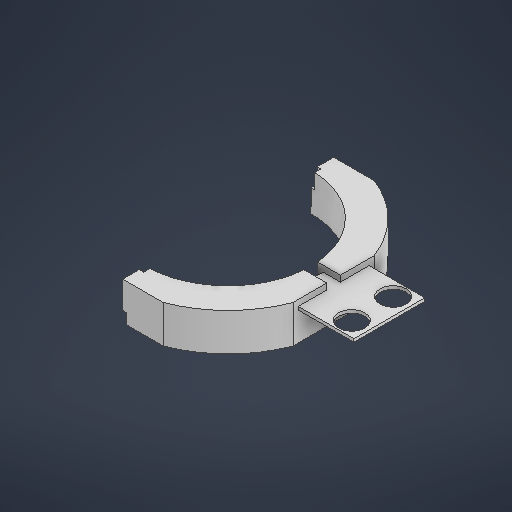
# Autodesk Inventor part: Kruh
Saved by Autodesk Inventor 2026.2 (Build 302298000, 298)
## iProperties
Created: 2026-03-13
Part Number: Kruh
Material: Všeobecné
Document SubType Name: Modeling
Designer: cerna
Density: 1 g/cm^3
Appearance: Výchozí
Author: cerna
Autodesk Inventor part; units mm, degrees
sketch "Náčrt1" plane through (0, 0, 0) normal (0, 1, 0) x (-1, 0, 0)
  circle A0 centre (0, 0) radius 55
  line L0 (0, -70) -> (26.9258, -70)
  line L1 (0, -70) -> (-26.9258, -70)
  line L2 (-70, 0) -> (-70, -26.9258)
  line L3 (-70, 0) -> (-70, 26.9258)
  line L4 (70, 0) -> (70, -26.9258)
  line L5 (70, 0) -> (70, 26.9258)
  line L6 (0, 70) -> (26.9258, 70)
  line L7 (0, 70) -> (-26.9258, 70)
  line L8 (-104.3981, 0) -> (104.3981, 0) projected
  line L9 (0, -104.3981) -> (0, 104.3981) projected
  arc A1 (26.9258, -70) -> (70, -26.9258) centre (0, 0) ccw
  arc A2 (-70, -26.9258) -> (-26.9258, -70) centre (0, 0) ccw
  arc A3 (70, 26.9258) -> (26.9258, 70) centre (0, 0) ccw
  arc A4 (-26.9258, 70) -> (-70, 26.9258) centre (0, 0) ccw
  dimension "d1" = 110
  constraints: 16 end point, 8 point on circle, 7 parallel, 5 centre point, 2 coincident, 2 point on line, 1 perpendicular
  measures "d1" diameter of A0
extrude "Vysunutí1" add sketch "Náčrt1" along normal blind 25 contours L8 L4 A1 L0 L9 A0 | A0 L9 L6 A3 L5 L8 | A0 L8 L3 A4 L7 L9 | L9 L1 A2 L2 L8 A0
sketch "Náčrt2" plane through (-26.9258, 0, 70) normal (0, 0, 1) x (1, 0, 0)
  line L0 (53.8516, 0) -> (0, 0) projected
  line L1 (24.4258, 0) -> (29.4258, 0)
  line L2 (29.4258, 0) -> (29.4258, 7)
  line L3 (29.4258, 7) -> (24.4258, 7)
  line L4 (24.4258, 7) -> (24.4258, 0)
  line L5 (96.9258, 0) -> (96.9258, 25) projected
  point P0 (26.9258, 0)
  dimension "d5" = 5
  dimension "d6" = 7
  dimension "d7" = 67.5
  constraints: 8 end point, 2 parallel, 1 horizontal, 1 perpendicular, 1 point on line
  measures "d5" distance of L3.end L2.end
  measures "d6" distance of L2.end L1.end
  measures "d7" distance between parallel lines of L5 L2
extrude "Vysunutí2" cut sketch "Náčrt2" against normal blind 4.5
sketch "Náčrt3" plane through (26.9258, 0, -70) normal (0, 0, -1) x (-1, 0, 0)
  line L0 (0, 0) -> (53.8516, 0) projected
  line L1 (53.8516, 0) -> (53.8516, 25) projected
  line L2 (0, 25) -> (53.8516, 25) projected
  line L3 (0, 0) -> (0, 25) projected
  line L4 (53.8516, 0) -> (96.9258, 0) projected
  line L5 (96.9258, 0) -> (96.9258, 25) projected
  line L6 (53.8516, 25) -> (96.9258, 25) projected
  line L7 (53.8516, 0) -> (53.8516, 25) projected
  line L8 (24.4258, 0) -> (0, 0) projected
  line L9 (24.4258, 0) -> (29.4258, 0)
  line L10 (29.4258, 0) -> (29.4258, 7)
  line L11 (29.4258, 7) -> (24.4258, 7)
  line L12 (24.4258, 7) -> (24.4258, 0)
  point P0 (26.9258, 0)
  dimension "d10" = 5
  dimension "d11" = 7
  dimension "d12" = 67.5
  constraints: 8 end point, 2 parallel, 1 horizontal, 1 perpendicular, 1 point on line
  measures "d10" distance of L11.end L10.end
  measures "d11" distance of L10.end L9.end
  measures "d12" distance between parallel lines of L5 L10
extrude "Vysunutí3" cut sketch "Náčrt3" against normal blind 4.5 contours L12 L11 L10 L0
sketch "Náčrt4" plane through (0, 25, 0) normal (0, 1, 0) x (1, 0, 0)
  line L0 (70, -26.9258) -> (70, 26.9258) projected
  line L1 (70, -4.5) -> (52.6737, -4.5)
  line L2 (52.6737, -4.5) -> (52.6737, 4.5)
  line L3 (52.6737, 4.5) -> (70, 4.5)
  line L4 (70, 4.5) -> (70, -4.5)
  line L5 (-98, 0) -> (98, 0) projected
  line L6 (0, 98) -> (0, -98) projected
  point P0 (0, 0)
  point P1 (70, 4.5)
  dimension "d15" = 9
  dimension "d16" = 4.5
  constraints: 8 end point, 2 parallel, 1 horizontal, 1 perpendicular, 1 point on line
  measures "d15" distance between parallel lines of L1 L3
  measures "d16" distance between parallel lines of L5 L1
extrude "Vysunutí4" cut sketch "Náčrt4" against normal blind 4
ref_plane "Pracovní rovina2" through (0, 0, 54.5) normal (0, 0, 1) x (1, 0, 0)
sketch "Náčrt6" plane through (0, 0, 54.5) normal (0, 0, 1) x (1, 0, 0)
  line L0 (-26.9258, 25) -> (26.9258, 25) projected
  line L1 (3, 25) -> (-3, 25)
  line L2 (-3, 25) -> (-3, 15)
  line L3 (-3, 15) -> (3, 15)
  line L4 (3, 15) -> (3, 25)
  line L5 (0, 30) -> (0, -5) projected
  point P0 (0, 0)
  dimension "d21" = 6
  dimension "d22" = 10
  constraints: 8 end point, 2 parallel, 1 horizontal, 1 perpendicular, 1 point on line, 1 other
  measures "d21" distance of L3.end L2.end
  measures "d22" distance of L2.end L1.end
extrude "Vysunutí5" cut sketch "Náčrt6" along normal blind 4.5
ref_plane "Pracovní rovina3" through (0, 0, -54.5) normal (0, 0, 1) x (1, 0, 0)
sketch "Náčrt7" plane through (0, 0, -54.5) normal (0, 0, 1) x (1, 0, 0)
  line L0 (-55, 25) -> (54.8156, 25) projected
  line L1 (2.5, 25) -> (-2.5, 25)
  line L2 (-2.5, 25) -> (-2.5, 15)
  line L3 (-2.5, 15) -> (2.5, 15)
  line L4 (2.5, 15) -> (2.5, 25)
  line L5 (0, 30) -> (0, -5) projected
  point P0 (0, 0)
  point P1 (-3, 25)
  dimension "d26" = 5
  dimension "d27" = 10
  constraints: 8 end point, 2 parallel, 1 horizontal, 1 perpendicular, 1 point on line, 1 other
  measures "d26" distance of L3.end L2.end
  measures "d27" distance of L2.end L1.end
extrude "Vysunutí6" cut sketch "Náčrt7" against normal blind 4.5
sketch "Náčrt8" plane through (70, 0, 26.9258) normal (1, 0, 0) x (0, 0, -1)
  line L0 (3.4258, 21) -> (50.4258, 21)
  line L1 (50.4258, 21) -> (50.4258, 19)
  line L2 (50.4258, 19) -> (3.4258, 19)
  line L3 (3.4258, 19) -> (3.4258, 21)
  line L4 (31.4258, 21) -> (22.4258, 21) projected
  line L5 (53.8516, 25) -> (0, 25) projected
  line L6 (26.9258, 25) -> (26.9258, 9.9917)
  point P0 (26.9258, 0)
  dimension "d30" = 47
  dimension "d31" = 2
  constraints: 10 end point, 2 parallel, 1 collinear, 1 horizontal, 1 midpoint, 1 perpendicular, 1 vertical, 1 other
  measures "d30" distance of L1.end L2.end
  measures "d31" distance of L2.end L0.start
extrude "Vysunutí7" add sketch "Náčrt8" along normal blind 37
sketch "Náčrt9" plane through (0, 21, 0) normal (0, 1, 0) x (1, 0, 0)
  circle A0 centre (95.75, -13.75) radius 8.75
  circle A1 centre (95.75, 13.75) radius 8.75
  line L0 (-105.4, 0) -> (142.4, 0) projected
  line L1 (107, 23.5) -> (107, -23.5) projected
  point P0 (0, 0)
  dimension "d34" = 17.5
  dimension "d35" = 17.5
  dimension "d37" = 5
  dimension "d38" = 5
  dimension "d41" = 11.25
  dimension "d42" = 11.25
  constraints: 2 centre point
  measures "d34" diameter of A0
  measures "d35" diameter of A1
  measures "d37" distance edge to line of A1 L0
  measures "d38" distance edge to line of A0 L0
  measures "d41" distance from line of L1 A0.centre
  measures "d42" distance from line of L1 A1.centre
extrude "Vysunutí8" cut sketch "Náčrt9" against normal blind 27
ref_plane "Pracovní rovina4" through (54.5, 0, 0) normal (1, 0, 0) x (0, 1, 0)
sketch "Náčrt10" plane through (54.5, 0, 0) normal (1, 0, 0) x (0, 1, 0)
  line L0 (0, 55) -> (0, -55) projected
  line L1 (21, -4.5) -> (0, -4.5)
  line L2 (0, -4.5) -> (0, 4.5)
  line L3 (0, 4.5) -> (21, 4.5)
  line L4 (21, 4.5) -> (21, -4.5)
  point P0 (0, 0)
  dimension "d44" = 9
  constraints: 8 end point, 2 parallel, 1 horizontal, 1 perpendicular, 1 point on line
  measures "d44" distance of L3.end L1.start
extrude "Vysunutí9" cut sketch "Náčrt10" along normal blind 4
